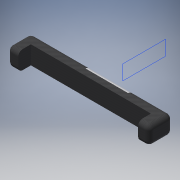
# Autodesk Inventor part: Bumper
Saved by Autodesk Inventor 2017 (Build 210142000, 142)
## iProperties
Created: 2018-01-27
Part Number: Bumper
Material: CFRP
Document SubType Name: Modeling
Designer: S331461152
Density: 1.43 g/cm^3
Appearance: Carbon Fiber
Author: S331461152
Autodesk Inventor part; units mm, degrees
ref_plane "YZ Plane" through (0, 0, 0) normal (1, 0, 0) x (0, 1, 0)
ref_plane "XZ Plane" through (0, 0, 0) normal (0, 1, 0) x (-1, 0, 0)
ref_plane "XY Plane" through (0, 0, 0) normal (0, 0, 1) x (1, 0, 0)
sketch "Sketch1" plane through (0, 0, 0) normal (0, 1, 0) x (-1, 0, 0)
  line L0 (0, 0) -> (-418.1447, 0)
  line L1 (-418.1447, 0) -> (-418.1447, -76.2)
  line L2 (-418.1447, -76.2) -> (0, -76.2)
  line L3 (0, -76.2) -> (0, 0)
  line L4 (0, -76.2) -> (76.2, -76.2)
  line L5 (76.2, -76.2) -> (76.2, 0)
  line L6 (76.2, 0) -> (0, 0)
  line L7 (0, 0) -> (0, -76.2)
  line L8 (0, 0) -> (76.2, 0)
  line L9 (76.2, 0) -> (76.2, 88.9)
  line L10 (76.2, 88.9) -> (0, 88.9)
  line L11 (0, 88.9) -> (0, 0)
  dimension "d0" = 418.1447
  dimension "d1" = 76.2
  dimension "d4" = 76.2
  dimension "d5" = 76.2
  dimension "d6" = 76.2
  dimension "d7" = 88.9
  constraints: 24 end point, 6 parallel, 3 horizontal, 3 perpendicular
  measures "d0" distance of L2.end L1.end
  measures "d1" distance of L1.end L0.end
  measures "d4" distance of L6.end L5.end
  measures "d5" distance of L5.end L4.end
  measures "d6" distance of L10.end L9.end
  measures "d7" distance of L9.end L8.end
extrude "Extrusion2" add sketch "Sketch1" along normal blind 127
mirror "Mirror1" about plane through (418.1447, 0, 0) normal (1, 0, 0) of "Extrusion2"
fillet "Fillet1" radius 31.75 8 edges at (-76.2, 127, 6.35) (-76.2, 0, 6.35) (418.1447, 127, -76.2) (418.1447, 0, -76.2) (-76.2, 63.5, -76.2) (912.4895, 63.5, -76.2) (912.4895, 127, 6.35) (912.4895, 0, 6.35)
fillet "Fillet2" radius 31.75 5 edges at (912.4895, 63.5, 88.9) (903.1901, 9.2994, 88.9) (858.5145, 0, 88.9) (858.5145, 127, 88.9) (903.1901, 117.7006, 88.9)
fillet "Fillet3" radius 31.75 5 edges at (-66.9006, 117.7006, 88.9) (-76.2, 63.5, 88.9) (-66.9006, 9.2994, 88.9) (-22.225, 0, 88.9) (-22.225, 127, 88.9)
sketch "Sketch3" plane through (880.7395, 31.75, -76.2) normal (0, 0, -1) x (-1, 0, 0)
  line L0 (314.0818, 85.8231) -> (611.0931, 85.8231) construction
  line L1 (611.0931, 85.8231) -> (611.0931, -17.1741) construction
  line L2 (611.0931, -17.1741) -> (314.0818, -17.1741) construction
  line L3 (314.0818, -17.1741) -> (314.0818, 85.8231) construction
  line L4 (925.1895, 63.5) -> (925.1895, 0) projected
  line L5 (0, 0) -> (0, 63.5) projected
  point P0 (880.7395, -31.75)
  dimension "d31" = 314.0964
  constraints: 2 other
  measures "d31" distance between parallel lines of L4 L1
decal "Decal1"
body "Solid2"
